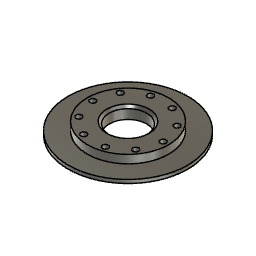
Load Plate (Autodesk Fusion 360 design; units mm, degrees)
Autodesk Fusion 360 part; units mm, degrees
sketch "Sketch1" plane through (0, 0, 0) normal (0, 0, 1) x (1, 0, 0)
  circle A0 centre (0, 0) radius 25.5
  dimension "d1" = 51
  constraint coincident A0.centre origin
  measures "d1" diameter of A0
extrude "Extrude1" add sketch "Sketch1" along normal blind 1.5
sketch "Sketch2" plane through (0, 0, 1.5) normal (0, 0, 1) x (-1, 0, 0)
  circle A0 centre (0, 0) radius 25.5
  circle A1 centre (0, 0) radius 17.35
  dimension "d4" = 34.7
  constraint coincident A0.centre A1.centre
  measures "d4" diameter of A1
extrude "Extrude2" add sketch "Sketch2" along normal blind 3.5 contours A1
sketch "Sketch3" plane through (0, 0, 5) normal (0, 0, 1) x (-1, 0, 0)
  circle A0 centre (0, 0) radius 17.35
  circle A1 centre (-15, 0) radius 1.25
  dimension "d8" = 2.5
  dimension "d9" = 15
  constraint horizontal A0.centre A1.centre
  measures "d8" diameter of A1
  measures "d9" distance of A0.centre A1.centre
extrude "Extrude3" cut sketch "Sketch3" against normal blind 20 contours A1
pattern_circular "C-Pattern1" count 10 over 360 about axis through (0, 0, 1.75) along (0, 0, 1) of "Extrude3"
sketch "Sketch4" plane through (0, 0, 5) normal (0, 0, 1) x (-1, 0, 0)
  circle A0 centre (-12.1353, 8.8168) radius 1.25
  circle A1 centre (-4.6353, 14.2658) radius 1.25
  circle A2 centre (4.6353, 14.2658) radius 1.25
  circle A3 centre (12.1353, 8.8168) radius 1.25
  circle A4 centre (15, 0) radius 1.25
  circle A5 centre (12.1353, -8.8168) radius 1.25
  circle A6 centre (4.6353, -14.2658) radius 1.25
  circle A7 centre (-4.6353, -14.2658) radius 1.25
  circle A8 centre (-12.1353, -8.8168) radius 1.25
  circle A9 centre (-15, 0) radius 1.25
  circle A10 centre (0, 0) radius 17.35
  circle A11 centre (0, 0) radius 8
  dimension "d14" = 16
  constraint coincident A10.centre A11.centre
  measures "d14" diameter of A11
extrude "Extrude4" cut sketch "Sketch4" against normal blind 20 contours A11
chamfer "Chamfer1" distance 1 angle 45 1 edges at (7.4586, -2.8929, 5)
sketch "Sketch5" plane through (0, 0, 5) normal (0, 0, 1) x (-1, 0, 0)
  circle A0 centre (0, 0) radius 17.35
  circle A1 centre (-15, 0) radius 1.25
  circle A2 centre (-12.1353, -8.8168) radius 1.25
  circle A3 centre (-4.6353, -14.2658) radius 1.25
  circle A4 centre (4.6353, -14.2658) radius 1.25
  circle A5 centre (12.1353, -8.8168) radius 1.25
  circle A6 centre (15, 0) radius 1.25
  circle A7 centre (12.1353, 8.8168) radius 1.25
  circle A8 centre (4.6353, 14.2658) radius 1.25
  circle A9 centre (-4.6353, 14.2658) radius 1.25
  circle A10 centre (-12.1353, 8.8168) radius 1.25
  circle A11 centre (0, 0) radius 9
equation "d4 = 35 mm - offset"
equation "offset = 0.3 mm"
